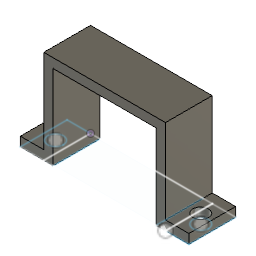
MixingStick_MotorHolder (Autodesk Fusion 360 design; units mm, degrees)
part number: 2026-05-26-16-55-25-903
Autodesk Fusion 360 part; units mm, degrees
note: some values were not read from the file. Set by a fixed rule: which sketch regions a step uses.
sketch "Sketch1" plane through (0, 0, 0) normal (0, 0, 1) x (1, 0, 0)
  line L0 (0, 0) -> (26, 0)
  line L1 (26, 0) -> (26, -10)
  line L2 (26, -10) -> (0, -10)
  line L3 (0, -10) -> (0, 0)
  line L4 (0, -10) -> (-5, -10)
  line L5 (-5, -10) -> (-5, 0)
  line L6 (-5, 0) -> (0, 0)
  line L7 (0, 0) -> (0, -10)
  line L8 (26, -10) -> (26, 0)
  circle A0 centre (-2.4667, -5) radius 1.65
  line L9 (26, 0) -> (31, 0)
  line L10 (31, 0) -> (31, -10)
  line L11 (31, -10) -> (26, -10)
  line L12 (26, -10) -> (26, 0)
  circle A1 centre (28.5333, -5) radius 1.65
  line L13 (2, -10) -> (24, -10)
  line L14 (24, -10) -> (24, 0)
  line L15 (24, 0) -> (2, 0)
  line L16 (2, 0) -> (2, -10)
  dimension "d1" = 10
  dimension "d2" = 26
  dimension "d7" = 3.3
  dimension "d11" = 3.3
  constraint horizontal L0
  constraint vertical L1
  constraint horizontal L2
  constraint vertical L3
  constraint coincident L0.start L3.end
  constraint horizontal L4
  constraint vertical L5
  constraint horizontal L6
  constraint vertical L7
  constraint vertical L8
  constraint horizontal L9
  constraint vertical L10
  constraint horizontal L11
  constraint vertical L12
  constraint horizontal L13
  constraint vertical L14
  constraint horizontal L15
  constraint vertical L16
  constraint coincident L0 L14.end
  constraint coincident L2 L13.start
  measures "d1" distance of L0.start L2.end
  measures "d2" distance of L0.start L0.end
  measures "d7" diameter of A0
  measures "d11" diameter of A1
extrude "Extrude1" add sketch "Sketch1" along normal blind 12 contours L0 L2 L3 L7 L16 | L0 L2 L13 L14 L15 L16 | L0 L1 L2 L8 L12 L14
extrude "Extrude2" add sketch "Sketch1" along normal blind 2 contours L3 L4 L5 L6 L7 | L0 L1 L2 L8 L12 L14 | A0
extrude "Extrude3" cut sketch "Sketch1" along normal blind 2 contours A0
extrude "Extrude4" add sketch "Sketch1" along normal blind 2 contours L1 L8 L9 L10 L11 L12
extrude "Extrude5" cut sketch "Sketch1" along normal blind 10 contours L0 L2 L13 L14 L15 L16
extrude "Extrude6" add 1 faces at (8.6667, -3.3333, 12) along direction (0, 0, 1) blind 10
extrude "Extrude7" cut 1 faces at (9.3333, -3.3333, 10) along direction (0, 0, 1) blind 8
extrude "Extrude8" cut 1 faces at (8.6667, -3.3333, 22) along direction (0, 0, -1) blind 2
